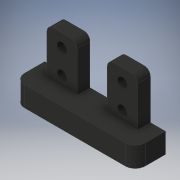
# Autodesk Inventor part: Heated Bed Belt Mount
Saved by Autodesk Inventor 2020.2 (Build 242310000, 310)
## iProperties
Created: 2019-05-18
Part Number: Heated Bed Belt Mount
Material: ABS Plastic
Document SubType Name: Modeling
Designer: Richard Hall
Density: 1.06 g/cm^3
Appearance: Rubber - Black
Author: Richard Hall
Autodesk Inventor part; units mm, degrees
ref_plane "YZ Plane" through (0, 0, 0) normal (1, 0, 0) x (0, 1, 0)
ref_plane "XZ Plane" through (0, 0, 0) normal (0, 1, 0) x (-1, 0, 0)
ref_plane "XY Plane" through (0, 0, 0) normal (0, 0, 1) x (1, 0, 0)
sketch "Sketch1" plane through (0, 0, 0) normal (0, 1, 0) x (-1, 0, 0)
  line L0 (25, 7.5) -> (-25, 7.5)
  line L1 (-30, 2.5) -> (-30, -7.5)
  line L2 (-30, -7.5) -> (30, -7.5)
  line L3 (30, -7.5) -> (30, 2.5)
  line L4 (30, 7.5) -> (-30, -7.5) construction
  line L5 (-30, 7.5) -> (30, -7.5) construction
  arc A0 (30, 2.5) -> (25, 7.5) centre (25, 2.5) ccw
  arc A1 (-25, 7.5) -> (-30, 2.5) centre (-25, 2.5) ccw
  point P0 (0, 0)
  dimension "d0" = 60
  dimension "d1" = 15
  dimension "d2" = 5
  constraints: 12 end point, 4 point on circle, 4 point on line, 4 tangent, 2 centre point, 2 midpoint, 2 parallel, 1 equal radius, 1 horizontal, 1 perpendicular
  measures "d0" distance of L1.end L2.end
  measures "d1" distance of L2.end L4.start
  measures "d2" radius of A0
extrude "Extrusion1" add sketch "Sketch1" along normal blind 10
sketch "Sketch2" plane through (0, 10, 0) normal (0, 1, 0) x (1, 0, 0)
  line L0 (7.5, 1.1) -> (22.5, 1.1)
  line L1 (22.5, 1.1) -> (22.5, 7.5)
  line L2 (22.5, 7.5) -> (7.5, 7.5)
  line L3 (7.5, 7.5) -> (7.5, 1.1)
  line L4 (7.5, 1.1) -> (22.5, 7.5) construction
  line L5 (22.5, 1.1) -> (7.5, 7.5) construction
  line L6 (30, -2.5) -> (30, 7.5) projected
  line L7 (30, 7.5) -> (-30, 7.5) projected
  point P0 (0, 0)
  point P1 (15, 4.3)
  dimension "d5" = 15
  dimension "d6" = 6.4
  dimension "d7" = 7.5
  constraints: 12 end point, 2 midpoint, 2 parallel, 1 collinear, 1 horizontal, 1 perpendicular
  measures "d5" distance of L2.end L1.end
  measures "d6" distance of L1.end L0.end
  measures "d7" distance between parallel lines of L6 L1
extrude "Extrusion2" add sketch "Sketch2" along normal blind 23
fillet "Fillet1" radius 3 2 edges at (7.5, 33, -4.3) (22.5, 33, -4.3)
sketch "Sketch3" plane through (30, 0, -7.5) normal (0, 0, -1) x (-1, 0, 0)
  arc A0 (10.5, 33) -> (7.5, 30) centre (10.5, 30) ccw projected
  line L0 (7.5, 10) -> (7.5, 30) projected
  line L1 (0, 10) -> (7.5, 10) projected
  line L2 (0, 0) -> (0, 10) projected
  line L3 (60, 0) -> (0, 0) projected
  line L4 (60, 0) -> (60, 10) projected
  line L5 (22.5, 10) -> (60, 10) projected
  line L6 (22.5, 10) -> (22.5, 30) projected
  arc A1 (22.5, 30) -> (19.5, 33) centre (19.5, 30) ccw projected
  line L7 (10.5, 33) -> (19.5, 33) projected
  point P0 (30, 0)
  point P1 (15, 26.5)
  point P2 (15, 14.5)
  point P3 (15, 33)
  dimension "d11" = 12
  dimension "d29" = 14.5
  constraints: 2 vertical alignment, 1 midpoint
  measures "d11" distance of point (15, 14.5) point (15, 26.5)
  measures "d29" distance from line of L3 point (15, 14.5)
hole "Hole1" at (15, 26.5, -7.5) at (15, 14.5, -7.5) direction (0, 0, -1) diameter 5.2 end through all start extended yes
mirror "Mirror1" about plane through (0, 0, 0) normal (1, 0, 0) of "Extrusion2", "Hole1", "Fillet1"
sketch "Sketch4" plane through (0, 0, 0) normal (0, -1, 0) x (1, 0, 0)
  line L0 (22.5, 0) -> (-22.5, 0) construction
  point P0 (0, 0)
  point P1 (0, 0)
  dimension "d21" = 45
  constraints: 3 coincident, 2 end point, 1 horizontal, 1 midpoint
  measures "d21" distance of L0.start L0.end
hole "Hole2" at (22.5, 0, 0) at (-22.5, 0, 0) direction (0, 1, 0) diameter 5.2 depth 6.4
body "Solid1"
